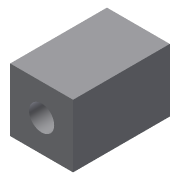
# Autodesk Inventor part: Screw Port 6_8
Saved by Autodesk Inventor 2016 (Build 200138000, 138)
## iProperties
Created: 2015-04-06
Part Number: Screw Port 6_8
Material: Generic
Document SubType Name: Modeling
Designer: Jonathan
Density: 1 g/cm^3
Appearance: Default
Author: Jonathan
Autodesk Inventor part; units mm, degrees
ref_plane "YZ Plane" through (0, 0, 0) normal (1, 0, 0) x (0, 1, 0)
ref_plane "XZ Plane" through (0, 0, 0) normal (0, 1, 0) x (-1, 0, 0)
ref_plane "XY Plane" through (0, 0, 0) normal (0, 0, 1) x (1, 0, 0)
sketch "Sketch1" plane through (0, 0, 0) normal (0, 1, 0) x (-1, 0, 0)
  line L0 (14.4237, 0) -> (-15, 0)
  line L1 (0, 25) -> (0, -25.6825)
  line L2 (6.5, 6.5) -> (-6.5, 6.5)
  line L3 (-6.5, 6.5) -> (-6.5, -6.5)
  line L4 (-6.5, -6.5) -> (6.5, -6.5)
  line L5 (6.5, -6.5) -> (6.5, 6.5)
  point P0 (0, 0)
  dimension "d0" = 13
  dimension "d1" = 0
  dimension "d10" = 0
  constraints: 12 end point, 2 parallel, 2 perpendicular, 1 horizontal, 1 vertical, 2 other
  measures "d0" distance of L3.end L4.end
  measures "d1" distance from line of point (0, 0) L0
  measures "d10" distance from line of point (0, 0) L1
extrude "Body" add sketch "Sketch1" along normal blind 20
sketch "Sketch2" plane through (0, 0, 0) normal (0, -1, 0) x (1, 0, 0)
  circle A0 centre (0, 0) radius 2.6
  dimension "d4" = 5.2
  constraints: 1 centre point, 1 coincident
  measures "d4" diameter of A0
extrude "Screw Thread Hole" cut sketch "Sketch2" against normal through all
sketch "Sketch3" plane through (0, 20, 0) normal (0, 1, 0) x (1, 0, 0)
  line L0 (4.25, -4.25) -> (-4.25, -4.25)
  line L1 (-4.25, -4.25) -> (-4.25, 4.25)
  line L2 (-4.25, 4.25) -> (4.25, 4.25)
  line L3 (4.25, 4.25) -> (4.25, -4.25)
  line L4 (4.25, -4.25) -> (-4.25, 4.25) construction
  line L5 (-4.25, -4.25) -> (4.25, 4.25) construction
  point P0 (0, 0)
  dimension "d11" = 8.5
  constraints: 12 end point, 2 midpoint, 2 parallel, 2 perpendicular, 1 horizontal
  measures "d11" distance of L1.end L2.end
extrude "Connector" cut sketch "Sketch3" against normal blind 6
body "Solid1"
